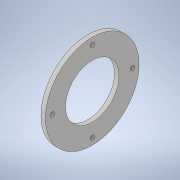
# Autodesk Inventor part: BearingAdapter
Saved by Autodesk Inventor 2021 (Build 250183000, 183)
## iProperties
Created: 2020-09-20
Part Number: BearingAdapter
Material: Generic
Document SubType Name: Modeling
Designer: PhotonUser
Density: 1 g/cm^3
Appearance: Default
Author: PhotonUser
Autodesk Inventor part; units mm, degrees
ref_plane "YZ Plane" through (0, 0, 0) normal (1, 0, 0) x (0, 1, 0)
ref_plane "XZ Plane" through (0, 0, 0) normal (0, 1, 0) x (-1, 0, 0)
ref_plane "XY Plane" through (0, 0, 0) normal (0, 0, 1) x (1, 0, 0)
sketch "Sketch3" plane through (0, 0, 0) normal (1, 0, 0) x (0, 1, 0)
  circle A0 centre (0, 0) radius 66.675
  circle A1 centre (0, -57.15) radius 3.175
  circle A2 centre (57.15, 0) radius 3.175
  circle A3 centre (0, 57.15) radius 3.175
  circle A4 centre (-57.15, 0) radius 3.175
  line L0 (0, 0) -> (79.9058, 0)
  circle A5 centre (0, 0) radius 38.1
  dimension "d13" = 133.35
  dimension "d14" = 6.35
  dimension "d17" = 360
  dimension "d19" = 57.15
  dimension "d20" = 76.2
  constraints: 6 centre point, 2 coincident, 2 end point, 1 horizontal, 1 point on line, 9 other
  measures "d13" diameter of A0
  measures "d14" diameter of A1
  measures "d19" distance of A1.centre point (0, 0)
  measures "d20" diameter of A5
extrude "Extrusion3" add sketch "Sketch3" along normal blind 6.35
body "Solid2"
